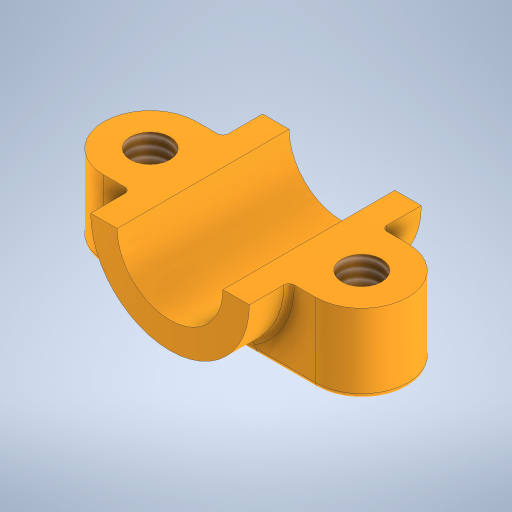
# Autodesk Inventor part: Thanh Truyen 1
Saved by Autodesk Inventor 2023 (Build 270158000, 158)
## iProperties
Created: 2023-10-06
Part Number: Thanh Truyen 1
Material: Generic
Document SubType Name: Modeling
Designer: huy20
Density: 1 g/cm^3
Appearance: Default
Author: huy20
Autodesk Inventor part; units mm, degrees
ref_plane "YZ Plane" through (0, 0, 0) normal (1, 0, 0) x (0, 1, 0)
ref_plane "XZ Plane" through (0, 0, 0) normal (0, 1, 0) x (-1, 0, 0)
sketch "Sketch1" plane through (0, 0, 0) normal (0, 1, 0) x (-1, 0, 0)
  arc A0 (-2, 0) -> (2, 0) centre (0, 0) ccw
  arc A1 (-3, 0) -> (3, 0) centre (0, 0) ccw
  line L0 (3, 0) -> (2, 0)
  line L1 (-2, 0) -> (-3, 0)
  dimension "d0" = 4
  dimension "d1" = 6
  constraints: 4 end point, 4 point on circle, 2 centre point, 2 coincident, 2 horizontal
  measures "d0" diameter of A0
  measures "d1" diameter of A1
extrude "Extrusion1" add sketch "Sketch1" along normal mid plane 6.5
ref_plane "Work Plane1" through (-3, 3.25, -3) normal (0, 0, 1) x (1, 0, 0)
sketch "Sketch2" plane through (-3, 3.25, -3) normal (0, 0, 1) x (1, 0, 0)
  line L0 (-1, -3.25) -> (7, -3.25) construction
  arc A0 (7, -5) -> (7, -1.5) centre (7, -3.25) ccw
  arc A1 (-1, -1.5) -> (-1, -5) centre (-1, -3.25) ccw
  line L1 (-1, -5) -> (7, -5)
  line L2 (-1, -1.5) -> (7, -1.5)
  line L3 (0, 0) -> (0, -6.5) projected
  point P0 (3, -3.25)
  dimension "d5" = 3.5
  dimension "d6" = 3.5
  dimension "d7" = 4
  dimension "d8" = 4
  dimension "d10" = 0
  constraints: 6 end point, 4 point on circle, 2 centre point, 2 coincident, 2 horizontal, 2 tangent, 1 perpendicular
  measures "d5" diameter of A0
  measures "d6" diameter of A1
  measures "d7" distance of point (3, -3.25) L0.end
  measures "d8" distance of L0.start point (3, -3.25)
  measures "d10" distance from line of point (3, -3.25) L0
extrude "Extrusion2" add sketch "Sketch2" along normal up to surface (3 mm away)
sketch "Sketch3" plane through (0, 0, 0) normal (0, 1, 0) x (-1, 0, 0)
  arc A0 (-2, 0) -> (2, 0) centre (0, 0) ccw projected
  line L0 (2, 0) -> (-2, 0) projected
  circle A1 centre (0, 0) radius 2
  constraints: 1 centre point, 1 coincident
extrude "Extrusion3" cut sketch "Sketch3" along normal mid plane 10 contours L0 A0
sketch "Sketch4" plane through (-3, 3.25, -3) normal (0, 0, -1) x (-1, 0, 0)
  arc A0 (-7, -1.5) -> (-7, -5) centre (-7, -3.25) ccw projected
  point P0 (-3, -3.25)
  point P1 (1, -3.25)
  constraints: 1 coincident
hole "Hole1" at (-4, 0, -3) at (4, 0, -3) direction (0, 0, 1) diameter 1.5 end through all
thread "Thread1" size "M1.6x0.35" class "6H" standard "ANSI Metric M Profile" length 21
thread "Thread2" size "M1.6x0.35" class "6H" standard "ANSI Metric M Profile" length 21
fillet "Fillet1" radius 0.2 10 edges at (2.1213, -1.75, -2.1213) (-2.1213, -1.75, -2.1213) (-5.75, 0, -3) (-2, 1.75, -3) (-2, -1.75, -3) (5.75, 0, -3) (2, 1.75, -3) (2, -1.75, -3) (2.1213, 1.75, -2.1213) (-2.1213, 1.75, -2.1213)
body "Solid1"
